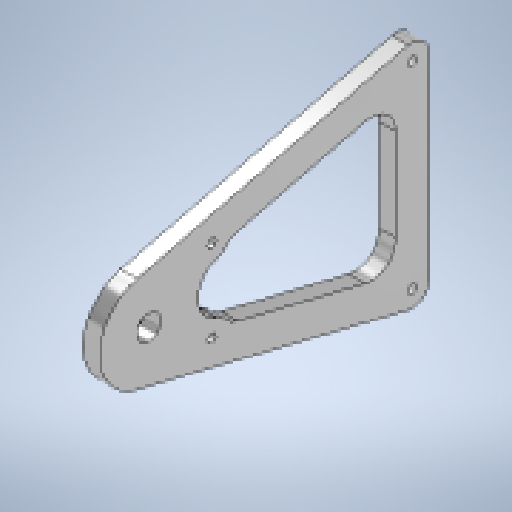
# Autodesk Inventor part: Frame (Motor Side)
Saved by Autodesk Inventor 2023 (Build 270158000, 158)
## iProperties
Created: 2022-05-22
Part Number: Frame (Motor Side)
Material: Aluminum 6061
Document SubType Name: Modeling
Designer: Nathan Cai
Density: 2.7 g/cm^3
Appearance: Aluminum - Flat
Mass: 78.0401 g
Surface Area: 132.733 cm^2
Volume: 28.9038 cm^3
Leg_Mounts: 0.625 in
Leg_Offset: 0.750 in
C2C: 4.250 in
Author: Nathan Cai
Autodesk Inventor part; units mm, degrees
ref_plane "YZ Plane" through (0, 0, 0) normal (1, 0, 0) x (0, 1, 0)
ref_plane "XZ Plane" through (0, 0, 0) normal (0, 1, 0) x (-1, 0, 0)
ref_plane "XY Plane" through (0, 0, 0) normal (0, 0, 1) x (1, 0, 0)
sketch "Sketch1" plane through (0, 0, 0) normal (1, 0, 0) x (0, 1, 0)
  circle A0 centre (0, 0) radius 4.7625 construction
  line L0 (0, 0) -> (0, 107.95) construction
  circle A1 centre (0, 107.95) radius 4.7625
  circle A2 centre (0, 107.95) radius 76.2 construction
  circle A3 centre (0, 107.95) radius 19.05
  line L1 (0, 6.35) -> (38.1, 6.35) construction
  circle A4 centre (38.1, 6.35) radius 1.7526
  circle A5 centre (38.1, 6.35) radius 6.35
  line L2 (18.4974, 112.5053) -> (44.2658, 7.8684)
  line L3 (10.4605, 92.0289) -> (31.9342, 4.8316)
  circle A6 centre (-38.1, 6.35) radius 1.7526
  circle A7 centre (-38.1, 6.35) radius 6.35
  line L4 (-18.4974, 112.5053) -> (-44.2658, 7.8684)
  line L5 (-10.4605, 92.0289) -> (-31.9342, 4.8316)
  line L6 (38.1, 12.7) -> (-38.1, 12.7)
  line L7 (-38.1, 0) -> (38.1, 0)
  line L8 (38.1, 6.35) -> (15.7269, 97.1997) construction
  circle A8 centre (19.05, 83.7056) radius 1.7526
  circle A9 centre (-19.05, 83.7056) radius 1.7526
  line L9 (19.05, 83.7056) -> (-19.05, 83.7056) construction
  circle A10 centre (15.875, 83.7056) radius 6.35
  circle A11 centre (15.875, 83.7056) radius 1.7526
  circle A12 centre (-15.875, 83.7056) radius 6.35
  circle A13 centre (-15.875, 83.7056) radius 1.7526
  arc A14 (31.8736, 5.0775) -> (-32.2755, 0) centre (0, 0) ccw construction
  arc A15 (44.3636, 7.3939) -> (-44.3636, 7.3939) centre (0, 0) ccw construction
  point P0 (44.2067, 4.609)
  point P1 (-23.4623, 39.2331)
  point P2 (-18.4974, 112.5053)
  point P3 (-10.4605, 92.0289)
  point P4 (29.9965, 12.7)
  point P5 (-29.9965, 12.7)
  point P6 (-14.0047, 77.6373)
  point P7 (-11.4006, 88.2114)
  point P8 (11.4006, 88.2114)
  point P9 (14.0047, 77.6373)
  point P10 (23.7126, 38.2166)
  point P11 (-23.7126, 38.2166)
  point P12 (-42.8017, 13.8134)
  point P13 (-44.3636, 7.3939)
  point P14 (-31.8364, 5.3061)
  point P15 (31.8364, 5.3061)
  point P16 (44.3636, 7.3939)
  point P17 (42.8017, 13.8134)
  point P18 (-30.5865, 10.3042)
  point P19 (31.8736, 5.0775)
  point P20 (-31.8736, 5.0775)
  point P21 (30.5865, 10.3042)
  dimension "d0" = 9.525
  dimension "C2C" = 107.95
  dimension "d3" = 9.525
  dimension "d4" = 152.4
  dimension "d5" = 38.1
  dimension "d6" = 38.1
  dimension "d7" = 3.5052
  dimension "d8" = 12.7
  dimension "d9" = 6.35
  dimension "d10" = 12.7
  dimension "d37" = 3.5052
  dimension "Leg_Offset" = 19.05
  dimension "d39" = 12.7
  dimension "d40" = 3.5052
  dimension "Leg_Mounts" = 15.875
  dimension "d42" = 12.7
  constraints: 20 end point, 18 point on circle, 16 centre point, 11 coincident, 10 symmetric about line, 7 tangent, 6 point on line, 2 horizontal, 2 parallel, 1 vertical, 5 other
  measures "d0" diameter of A0
  measures "C2C" distance of L0.start L0.end
  measures "d3" diameter of A1
  measures "d4" diameter of A2
  measures "d5" diameter of A3
  measures "d6" distance of L1.start L1.end
  measures "d7" diameter of A4
  measures "d8" diameter of A5
  measures "d9" distance from line of A0.centre L1
  measures "d10" distance between parallel lines of L2 L3
  measures "d37" diameter of A8
  measures "Leg_Offset" distance from line of L0 L9.start
  measures "d39" diameter of A10
  measures "d40" diameter of A11
  measures "Leg_Mounts" distance from line of L0 A11.centre
  measures "d42" radial gap between concentric circles of A14 A15
extrude "Extrusion1" add sketch "Sketch1" along normal blind 6.35 contours A3 | A3 L2 A5 L6 L3 A10 | A3 L5 A12 L6 A7 L4 | A5 | A10 L3 | L3 A10 | A7 | A5 L3 L6 | A12 L5 | L5 A12 | L6 L5 A7 | A7 L5 L6 L3 A5 L7 | A8 A11 | A13 A9 picked at (19.7267, 83.5634) picked at (-19.7267, 83.8478)
fillet "Fillet1" radius 9.525 8 edges at (3.175, 10.4605, 92.0289) (3.175, -10.4605, 92.0289) (3.175, 14.0047, 77.6373) (3.175, -14.0047, 77.6373) (3.175, 11.4006, 88.2114) (3.175, -11.4006, 88.2114) (3.175, 29.9965, 12.7) (3.175, -29.9965, 12.7)
fillet "Fillet2" [suppressed]
equation "\"d10\" = d8"
body "Solid1"
